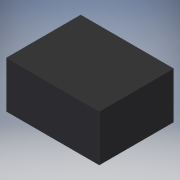
# Autodesk Inventor part: Falange-media
Saved by Autodesk Inventor 2018 (Build 220112000, 112)
## iProperties
Created: 2017-06-03
Part Number: Falange-media
Material: Genérico
Document SubType Name: Modeling
Designer: Vitor
Density: 1 g/cm^3
Appearance: Padrão
Author: Vitor
Autodesk Inventor part; units mm, degrees
ref_plane "YZ Plane" through (0, 0, 0) normal (1, 0, 0) x (0, 1, 0)
ref_plane "XZ Plane" through (0, 0, 0) normal (0, 1, 0) x (-1, 0, 0)
ref_plane "XY Plane" through (0, 0, 0) normal (0, 0, 1) x (1, 0, 0)
sketch "Esboço1" plane through (0, 0, 0) normal (0, 0, 1) x (1, 0, 0)
  line L0 (0, 0) -> (21, 0)
  line L1 (21, 0) -> (21, -21)
  line L2 (21, -21) -> (0, -21)
  line L3 (0, -21) -> (0, 0)
  dimension "d0" = 21
  dimension "d1" = 21
  constraints: 8 end point, 3 perpendicular, 1 horizontal
  measures "d0" distance of L0.start L0.end
  measures "d1" distance of L0.end L1.end
extrude "Extrusão1" add sketch "Esboço1" along normal blind 30
sketch "Esboço4" plane through (0, 0, 0) normal (0, 0, -1) x (-1, 0, 0)
  line L0 (-21, -21) -> (0, -21) projected
  line L1 (-21, -21) -> (0, -21)
  line L2 (0, -21) -> (0, 0)
  line L3 (0, 0) -> (-21, 0)
  line L4 (-21, 0) -> (-21, -21)
  constraints: 8 end point, 2 parallel, 1 horizontal, 1 perpendicular
extrude "Extrusão4" cut sketch "Esboço4" against normal blind 10
sketch "Esboço5" plane through (0, 0, 10) normal (0, 0, -1) x (-1, 0, 0)
  line L0 (-15, -21) -> (-21, -21) projected
  line L1 (-21, -21) -> (0, -21)
  line L2 (0, -21) -> (0, 0)
  line L3 (0, 0) -> (-21, 0)
  line L4 (-21, 0) -> (-21, -21)
  constraints: 8 end point, 2 parallel, 1 horizontal, 1 perpendicular
extrude "Extrusão5" cut sketch "Esboço5" against normal blind 10
sketch "Esboço14" plane through (0, 0, 20) normal (0, 0, -1) x (-1, 0, 0)
  line L0 (-21, -21) -> (-21, 0) projected
  line L1 (-21, -21) -> (-21, -16)
  line L2 (-21, -16) -> (0, -16)
  line L3 (0, 0) -> (0, -21) projected
  line L4 (0, -16) -> (0, -21)
  line L5 (0, -21) -> (-21, -21) projected
  line L6 (0, -21) -> (-21, -21)
  line L7 (-21, -21) -> (0, -21)
  line L8 (0, -21) -> (-1, -21)
  line L9 (-1, -21) -> (-1, 0)
  line L10 (-21, 0) -> (0, 0) projected
  line L11 (-1, 0) -> (0, 0)
  line L12 (0, 0) -> (0, -21)
  line L13 (-1, -21) -> (-1, 0)
  line L14 (0, 0) -> (-1, 0)
  line L15 (0, 0) -> (-1, 0)
  line L16 (0, 0) -> (0, -21)
  line L17 (0, -21) -> (-1, -21)
  line L18 (-21, -21) -> (0, -21)
  line L19 (0, -21) -> (0, -16)
  line L20 (0, -16) -> (-21, -16)
  line L21 (-21, -16) -> (-21, -21)
  dimension "d45" = 5
  dimension "d46" = 1
  constraints: 36 end point, 7 collinear, 6 perpendicular, 2 parallel, 2 point on line, 1 horizontal
  measures "d45" distance of L0.start L1.end
  measures "d46" distance of L3.end L8.end
extrude "Extrusão14" cut sketch "Esboço14" against normal blind 30 contours L0 L2 L9 L5 | L9 L2 L3 L5 | L9 L10 L3 L2
